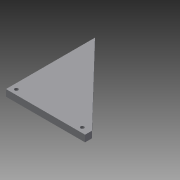
# Autodesk Inventor part: BallGuidePly
Saved by Autodesk Inventor 2014 (Build 180170000, 170)
## iProperties
Created: 2016-02-08
Part Number: BallGuidePly
Material: Generic
Document SubType Name: Modeling
Designer: choices
Density: 1 g/cm^3
Appearance: Default
Author: choices
Autodesk Inventor part; units mm, degrees
ref_plane "YZ Plane" through (0, 0, 0) normal (1, 0, 0) x (0, 1, 0)
ref_plane "XZ Plane" through (0, 0, 0) normal (0, 1, 0) x (-1, 0, 0)
ref_plane "XY Plane" through (0, 0, 0) normal (0, 0, 1) x (1, 0, 0)
sketch "Sketch1" plane through (0, 0, 0) normal (0, 1, 0) x (-1, 0, 0)
  line L0 (-91.7523, 23.1497) -> (73.3477, 23.1497)
  line L1 (73.3477, 23.1497) -> (73.3477, -148.2749)
  line L2 (73.3477, -148.2749) -> (-91.7523, 23.1497)
  circle A0 centre (62.7836, 13.6247) radius 3.3528
  circle A1 centre (-64.2164, 13.6247) radius 3.3566
  line L3 (-79.0523, 23.1497) -> (-79.0523, 9.9632)
  point P0 (0, 0)
  dimension "d0" = 165.1
  dimension "d1" = 171.4246
  dimension "d2" = 6.7056
  dimension "d3" = 9.525
  dimension "d4" = 6.7132
  dimension "d5" = 127
  dimension "d8" = 12.7
  constraints: 8 end point, 2 centre point, 2 point on line, 1 horizontal, 1 parallel, 1 perpendicular
  measures "d0" distance of L0.start L0.end
  measures "d1" distance of L0.end L1.end
  measures "d2" diameter of A0
  measures "d3" distance from line of L0 A0.centre
  measures "d4" diameter of A1
  measures "d5" distance of A0.centre A1.centre
  measures "d8" distance from line of L3 L0.start
extrude "Extrusion1" add sketch "Sketch1" along normal blind 12.7 contours L0 L1 L2 L3
body "Solid1"
